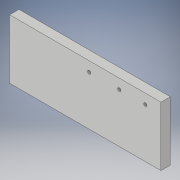
# Autodesk Inventor part: Kermit bumper Medium
Saved by Autodesk Inventor 2018 (Build 220112000, 112)
## iProperties
Created: 2018-02-13
Part Number: Kermit bumper Medium
Material: Generic
Document SubType Name: Modeling
Designer: kalra.rohan
Density: 1 g/cm^3
Appearance: Default
Author: kalra.rohan
Autodesk Inventor part; units mm, degrees
ref_plane "YZ Plane" through (0, 0, 0) normal (1, 0, 0) x (0, 1, 0)
ref_plane "XZ Plane" through (0, 0, 0) normal (0, 1, 0) x (-1, 0, 0)
ref_plane "XY Plane" through (0, 0, 0) normal (0, 0, 1) x (1, 0, 0)
sketch "Sketch1" plane through (0, 0, 0) normal (0, 0, 1) x (1, 0, 0)
  line L0 (0, 0) -> (369.57, 0)
  line L1 (369.57, 0) -> (369.57, -144.78)
  line L2 (369.57, -144.78) -> (0, -144.78)
  line L3 (0, -144.78) -> (0, 0)
  circle A0 centre (331.47, -24.13) radius 3.9179
  circle A1 centre (267.97, -24.13) radius 3.9243
  circle A2 centre (194.31, -24.13) radius 3.9243
  dimension "d0" = 369.57
  dimension "d1" = 144.78
  dimension "d2" = 7.8359
  dimension "d3" = 38.1
  dimension "d4" = 120.65
  dimension "d5" = 7.8486
  dimension "d6" = 120.65
  dimension "d7" = 63.5
  dimension "d8" = 7.8486
  dimension "d9" = 120.65
  dimension "d10" = 73.66
  constraints: 8 end point, 3 centre point, 2 parallel, 1 horizontal, 1 perpendicular
  measures "d0" distance between parallel lines of L1 L3
  measures "d1" distance between parallel lines of L2 L0
  measures "d2" diameter of A0
  measures "d3" distance from line of L1 A0.centre
  measures "d4" distance from line of A0.centre L2
  measures "d5" diameter of A1
  measures "d6" distance from line of L2 A1.centre
  measures "d7" distance of A0.centre A1.centre
  measures "d8" diameter of A2
  measures "d9" distance from line of A2.centre L2
  measures "d10" distance of A1.centre A2.centre
extrude "Extrusion1" add sketch "Sketch1" against normal blind 22.86
body "Solid1"
